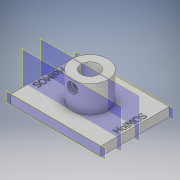
# Autodesk Inventor part: 1.3 Laserhalter_unten
Saved by Autodesk Inventor 2018.3 (Build 223284000, 284)
## iProperties
Created: 2018-11-22
Part Number: 1.3 Laserhalter_unten
Material: Generisch
Document SubType Name: Modeling
Designer: pgmadmin
Density: 1 g/cm^3
Appearance: Vorgabe
Author: pgmadmin
Autodesk Inventor part; units mm, degrees
ref_plane "YZ Plane" through (0, 0, 0) normal (1, 0, 0) x (0, 1, 0)
ref_plane "XY Plane" through (0, 0, 0) normal (0, 0, 1) x (1, 0, 0)
sketch "Skizze1" plane through (0, 0, 0) normal (0, 0, 1) x (1, 0, 0)
  line L0 (-25, -19) -> (25, -19)
  line L1 (25, -19) -> (25, 19)
  line L2 (25, 19) -> (-25, 19)
  line L3 (-25, 19) -> (-25, -19)
  line L4 (-25, -19) -> (25, 19) construction
  line L5 (25, -19) -> (-25, 19) construction
  point P0 (0, 0)
  dimension "d0" = 50
  dimension "d1" = 38
  constraints: 12 end point, 2 midpoint, 2 parallel, 1 horizontal, 1 perpendicular
  measures "d0" distance of L1.end L2.end
  measures "d1" distance of L0.end L1.end
extrude "Extrusion1" add sketch "Skizze1" along normal blind 5
sketch "Skizze2" plane through (0, 0, 5) normal (0, 0, 1) x (1, 0, 0)
  point P0 (0, 0)
ref_plane "Arbeitsebene1" through (0, 19, 0) normal (0, 1, 0) x (-1, 0, 0)
ref_plane "Arbeitsebene2" through (0, -19, 0) normal (0, 1, 0) x (-1, 0, 0)
sketch "Skizze4" plane through (0, 0, 5) normal (0, 0, 1) x (1, 0, 0)
  circle A0 centre (0, 0) radius 10
  circle A1 centre (0, 0) radius 5
  dimension "d12" = 20
  dimension "d13" = 10
  constraints: 2 centre point, 2 coincident
  measures "d12" diameter of A0
  measures "d13" diameter of A1
extrude "Extrusion2" add sketch "Skizze4" along normal blind 15
ref_plane "Arbeitsebene3" through (0, -10, 0) normal (0, 1, 0) x (-1, 0, 0)
sketch "Skizze5" plane through (0, -10, 0) normal (0, 1, 0) x (-1, 0, 0)
  line L0 (10, 20) -> (-10, 20) projected
  point P0 (0, 0)
  point P1 (0, 16)
  dimension "d17" = 4
  measures "d17" distance from line of point (0, 16) L0
hole "Bohrung1" at (0, -10, 16) direction (0, 1, 0) diameter 3 depth 8 tip angle 118 counterbore diameter 5.68 counterbore depth 2
sketch "Skizze6" plane through (0, -10, 0) normal (0, 1, 0) x (-1, 0, 0)
  point P0 (0, 0)
sketch "Skizze7" plane through (0, 0, 0) normal (0, 0, -1) x (-1, 0, 0)
  circle A0 centre (0, 0) radius 2.5
  dimension "d25" = 5
  constraints: 2 coincident, 1 centre point
  measures "d25" diameter of A0
hole "Bohrung2" at (0, 0, 0) direction (0, 0, 1) diameter 5 depth 5 tip angle 118
sketch "Skizze8" plane through (0, 0, 5) normal (0, 0, 1) x (1, 0, 0)
  line L0 (25, 19) -> (-25, 19) projected
  line L1 (-25, -19) -> (25, -19) projected
  line L2 (-24, 19) -> (24, 19)
  line L3 (24, 19) -> (24, -19)
  line L4 (24, -19) -> (-24, -19)
  line L5 (-24, -19) -> (-24, 19)
  line L6 (-25, 19) -> (-25, -19) projected
  line L7 (25, -19) -> (25, 19) projected
  line L8 (-24, 5.3865) -> (-24, 5.8517)
  line L9 (-24, 5.8517) -> (-22.2869, 5.8517)
  line L10 (-22.2869, 5.8517) -> (-22.2869, 7.4627)
  line L11 (-22.2869, 7.4627) -> (-24, 7.4627)
  line L12 (-24, 7.4627) -> (-24, 7.9279)
  line L13 (-24, 7.9279) -> (-20.5, 7.9279)
  line L14 (-20.5, 7.9279) -> (-20.5, 7.4627)
  line L15 (-20.5, 7.4627) -> (-21.8728, 7.4627)
  line L16 (-21.8728, 7.4627) -> (-21.8728, 5.8517)
  line L17 (-21.8728, 5.8517) -> (-20.5, 5.8517)
  line L18 (-20.5, 5.8517) -> (-20.5, 5.3865)
  line L19 (-20.5, 5.3865) -> (-24, 5.3865)
  spline S0 degree 2 poles (-22.6868, 2.5531) (-23.3505, 2.5531) (-24.0737, 3.1912) (-24.0737, 3.7245) knots 0 0 0 1 2 2 2
  spline S1 degree 2 poles (-24.0737, 3.7245) (-24.0737, 4.2719) (-23.3278, 4.8987) (-22.6868, 4.8987) knots 0 0 0 1 2 2 2
  spline S2 degree 2 poles (-22.6868, 4.8987) (-22.0288, 4.8987) (-21.2998, 4.252) (-21.2998, 3.7245) knots 0 0 0 1 2 2 2
  spline S3 degree 2 poles (-21.2998, 3.7245) (-21.2998, 3.1912) (-22.0259, 2.5531) (-22.6868, 2.5531) knots 0 0 0 1 2 2 2
  spline S4 degree 2 poles (-22.6868, 3.0097) (-22.1763, 3.0097) (-21.6799, 3.3813) (-21.6799, 3.7245) knots 0 0 0 1 2 2 2
  spline S5 degree 2 poles (-21.6799, 3.7245) (-21.6799, 4.0677) (-22.1763, 4.4421) (-22.6868, 4.4421) knots 0 0 0 1 2 2 2
  spline S6 degree 2 poles (-22.6868, 4.4421) (-23.1831, 4.4421) (-23.6937, 4.0677) (-23.6937, 3.7245) knots 0 0 0 1 2 2 2
  spline S7 degree 2 poles (-23.6937, 3.7245) (-23.6937, 3.3841) (-23.1917, 3.0097) (-22.6868, 3.0097) knots 0 0 0 1 2 2 2
  line L20 (-24, 1.6483) -> (-24, 2.0908)
  line L21 (-24, 2.0908) -> (-20.344, 2.0908)
  line L22 (-20.344, 2.0908) -> (-20.344, 1.6483)
  line L23 (-20.344, 1.6483) -> (-24, 1.6483)
  line L24 (-24, -2.0361) -> (-24, -1.5709)
  line L25 (-24, -1.5709) -> (-20.985, -1.5709)
  line L26 (-20.985, -1.5709) -> (-23.0357, -0.6576)
  line L27 (-23.0357, -0.6576) -> (-23.0357, -0.374)
  line L28 (-23.0357, -0.374) -> (-20.985, 0.5308)
  line L29 (-20.985, 0.5308) -> (-24, 0.5308)
  line L30 (-24, 0.5308) -> (-24, 0.9648)
  line L31 (-24, 0.9648) -> (-20.5, 0.9648)
  line L32 (-20.5, 0.9648) -> (-20.5, 0.3294)
  line L33 (-20.5, 0.3294) -> (-22.4485, -0.5442)
  line L34 (-22.4485, -0.5442) -> (-20.5, -1.3894)
  line L35 (-20.5, -1.3894) -> (-20.5, -2.0361)
  line L36 (-20.5, -2.0361) -> (-24, -2.0361)
  spline S8 degree 2 poles (-20.8999, -5.2212) (-21.1325, -5.4198) (-21.8132, -5.641) (-22.25, -5.641) knots 0 0 0 1 2 2 2
  spline S9 degree 2 poles (-22.25, -5.641) (-22.6754, -5.641) (-23.3647, -5.4254) (-23.5972, -5.2212) knots 0 0 0 1 2 2 2
  spline S10 degree 2 poles (-23.5972, -5.2212) (-23.8412, -5.0057) (-24.0737, -4.4356) (-24.0737, -4.0924) knots 0 0 0 1 2 2 2
  spline S11 degree 2 poles (-24.0737, -4.0924) (-24.0737, -3.7378) (-23.8327, -3.1706) (-23.5972, -2.9635) knots 0 0 0 1 2 2 2
  spline S12 degree 2 poles (-23.5972, -2.9635) (-23.3647, -2.7622) (-22.6811, -2.5466) (-22.25, -2.5466) knots 0 0 0 1 2 2 2
  spline S13 degree 2 poles (-22.25, -2.5466) (-21.8104, -2.5466) (-21.141, -2.765) (-20.8999, -2.9664) knots 0 0 0 1 2 2 2
  spline S14 degree 2 poles (-20.8999, -2.9664) (-20.6673, -3.1706) (-20.4263, -3.7407) (-20.4263, -4.0924) knots 0 0 0 1 2 2 2
  spline S15 degree 2 poles (-20.4263, -4.0924) (-20.4263, -4.4498) (-20.6759, -5.0227) (-20.8999, -5.2212) knots 0 0 0 1 2 2 2
  spline S16 degree 2 poles (-22.25, -5.156) (-21.904, -5.156) (-21.3679, -5.0057) (-21.1921, -4.8695) knots 0 0 0 1 2 2 2
  spline S17 degree 2 poles (-21.1921, -4.8695) (-21.0105, -4.7305) (-20.829, -4.3391) (-20.829, -4.0952) knots 0 0 0 1 2 2 2
  spline S18 degree 2 poles (-20.829, -4.0952) (-20.829, -3.8428) (-21.0049, -3.4627) (-21.1921, -3.3181) knots 0 0 0 1 2 2 2
  spline S19 degree 2 poles (-21.1921, -3.3181) (-21.3707, -3.1791) (-21.9096, -3.0316) (-22.25, -3.0316) knots 0 0 0 1 2 2 2
  spline S20 degree 2 poles (-22.25, -3.0316) (-22.9392, -3.0316) (-23.671, -3.6102) (-23.671, -4.0952) knots 0 0 0 1 2 2 2
  spline S21 degree 2 poles (-23.671, -4.0952) (-23.671, -4.5802) (-22.9392, -5.156) (-22.25, -5.156) knots 0 0 0 1 2 2 2
  spline S22 degree 2 poles (-24.0624, -7.1272) (-24.0624, -6.7472) (-23.9036, -6.2139) (-23.7901, -5.9785) knots 0 0 0 1 2 2 2
  line L37 (-23.7901, -5.9785) -> (-23.2058, -5.9785)
  line L38 (-23.2058, -5.9785) -> (-23.2058, -6.0126)
  spline S23 degree 2 poles (-23.2058, -6.0126) (-23.4214, -6.2423) (-23.6596, -6.8237) (-23.6596, -7.0932) knots 0 0 0 1 2 2 2
  spline S24 degree 2 poles (-23.6596, -7.0932) (-23.6596, -7.4789) (-23.3391, -7.8732) (-23.0754, -7.8732) knots 0 0 0 1 2 2 2
  spline S25 degree 2 poles (-23.0754, -7.8732) (-22.8655, -7.8732) (-22.6045, -7.6661) (-22.5393, -7.4421) knots 0 0 0 1 2 2 2
  spline S26 degree 2 poles (-22.5393, -7.4421) (-22.4939, -7.2804) (-22.4315, -7.0109) (-22.3805, -6.8096) knots 0 0 0 1 2 2 2
  spline S27 degree 2 poles (-22.3805, -6.8096) (-22.3323, -6.628) (-22.1876, -6.3416) (-22.0713, -6.231) knots 0 0 0 1 2 2 2
  spline S28 degree 2 poles (-22.0713, -6.231) (-21.955, -6.1232) (-21.643, -6.0041) (-21.4388, -6.0041) knots 0 0 0 1 2 2 2
  spline S29 degree 2 poles (-21.4388, -6.0041) (-21.0134, -6.0041) (-20.4376, -6.6677) (-20.4376, -7.1811) knots 0 0 0 1 2 2 2
  spline S30 degree 2 poles (-20.4376, -7.1811) (-20.4376, -7.4761) (-20.5539, -7.998) (-20.6645, -8.222) knots 0 0 0 1 2 2 2
  line L39 (-20.6645, -8.222) -> (-21.2204, -8.222)
  line L40 (-21.2204, -8.222) -> (-21.2204, -8.188)
  spline S31 degree 2 poles (-21.2204, -8.188) (-21.0673, -8.0207) (-20.8404, -7.4988) (-20.8404, -7.2123) knots 0 0 0 1 2 2 2
  spline S32 degree 2 poles (-20.8404, -7.2123) (-20.8404, -6.889) (-21.1438, -6.4891) (-21.3906, -6.4891) knots 0 0 0 1 2 2 2
  spline S33 degree 2 poles (-21.3906, -6.4891) (-21.6118, -6.4891) (-21.8756, -6.7245) (-21.9352, -6.9457) knots 0 0 0 1 2 2 2
  spline S34 degree 2 poles (-21.9352, -6.9457) (-21.9749, -7.0932) (-22.077, -7.5215) (-22.1195, -7.6633) knots 0 0 0 1 2 2 2
  spline S35 degree 2 poles (-22.1195, -7.6633) (-22.2301, -8.0235) (-22.6754, -8.3582) (-23.0016, -8.3582) knots 0 0 0 1 2 2 2
  spline S36 degree 2 poles (-23.0016, -8.3582) (-23.2087, -8.3582) (-23.6058, -8.1908) (-23.7447, -8.0405) knots 0 0 0 1 2 2 2
  spline S37 degree 2 poles (-23.7447, -8.0405) (-23.8979, -7.8732) (-24.0624, -7.4477) (-24.0624, -7.1272) knots 0 0 0 1 2 2 2
  line L41 (24, -5.5814) -> (24, -6.0466)
  line L42 (24, -6.0466) -> (22.2869, -6.0466)
  line L43 (22.2869, -6.0466) -> (22.2869, -7.6576)
  line L44 (22.2869, -7.6576) -> (24, -7.6576)
  line L45 (24, -7.6576) -> (24, -8.1228)
  line L46 (24, -8.1228) -> (20.5, -8.1228)
  line L47 (20.5, -8.1228) -> (20.5, -7.6576)
  line L48 (20.5, -7.6576) -> (21.8728, -7.6576)
  line L49 (21.8728, -7.6576) -> (21.8728, -6.0466)
  line L50 (21.8728, -6.0466) -> (20.5, -6.0466)
  line L51 (20.5, -6.0466) -> (20.5, -5.5814)
  line L52 (20.5, -5.5814) -> (24, -5.5814)
  spline S38 degree 2 poles (22.6868, -2.748) (23.3505, -2.748) (24.0737, -3.3861) (24.0737, -3.9194) knots 0 0 0 1 2 2 2
  spline S39 degree 2 poles (24.0737, -3.9194) (24.0737, -4.4668) (23.3278, -5.0936) (22.6868, -5.0936) knots 0 0 0 1 2 2 2
  spline S40 degree 2 poles (22.6868, -5.0936) (22.0288, -5.0936) (21.2998, -4.4469) (21.2998, -3.9194) knots 0 0 0 1 2 2 2
  spline S41 degree 2 poles (21.2998, -3.9194) (21.2998, -3.3861) (22.0259, -2.748) (22.6868, -2.748) knots 0 0 0 1 2 2 2
  spline S42 degree 2 poles (22.6868, -3.2046) (22.1763, -3.2046) (21.6799, -3.5762) (21.6799, -3.9194) knots 0 0 0 1 2 2 2
  spline S43 degree 2 poles (21.6799, -3.9194) (21.6799, -4.2626) (22.1763, -4.637) (22.6868, -4.637) knots 0 0 0 1 2 2 2
  spline S44 degree 2 poles (22.6868, -4.637) (23.1831, -4.637) (23.6937, -4.2626) (23.6937, -3.9194) knots 0 0 0 1 2 2 2
  spline S45 degree 2 poles (23.6937, -3.9194) (23.6937, -3.579) (23.1917, -3.2046) (22.6868, -3.2046) knots 0 0 0 1 2 2 2
  line L53 (24, -1.8432) -> (24, -2.2857)
  line L54 (24, -2.2857) -> (20.344, -2.2857)
  line L55 (20.344, -2.2857) -> (20.344, -1.8432)
  line L56 (20.344, -1.8432) -> (24, -1.8432)
  line L57 (24, 1.8412) -> (24, 1.376)
  line L58 (24, 1.376) -> (20.985, 1.376)
  line L59 (20.985, 1.376) -> (23.0357, 0.4627)
  line L60 (23.0357, 0.4627) -> (23.0357, 0.1791)
  line L61 (23.0357, 0.1791) -> (20.985, -0.7257)
  line L62 (20.985, -0.7257) -> (24, -0.7257)
  line L63 (24, -0.7257) -> (24, -1.1596)
  line L64 (24, -1.1596) -> (20.5, -1.1596)
  line L65 (20.5, -1.1596) -> (20.5, -0.5243)
  line L66 (20.5, -0.5243) -> (22.4485, 0.3493)
  line L67 (22.4485, 0.3493) -> (20.5, 1.1945)
  line L68 (20.5, 1.1945) -> (20.5, 1.8412)
  line L69 (20.5, 1.8412) -> (24, 1.8412)
  spline S46 degree 2 poles (20.8999, 5.0263) (21.1325, 5.2249) (21.8132, 5.4461) (22.25, 5.4461) knots 0 0 0 1 2 2 2
  spline S47 degree 2 poles (22.25, 5.4461) (22.6754, 5.4461) (23.3647, 5.2306) (23.5972, 5.0263) knots 0 0 0 1 2 2 2
  spline S48 degree 2 poles (23.5972, 5.0263) (23.8412, 4.8108) (24.0737, 4.2407) (24.0737, 3.8975) knots 0 0 0 1 2 2 2
  spline S49 degree 2 poles (24.0737, 3.8975) (24.0737, 3.543) (23.8327, 2.9757) (23.5972, 2.7686) knots 0 0 0 1 2 2 2
  spline S50 degree 2 poles (23.5972, 2.7686) (23.3647, 2.5673) (22.6811, 2.3517) (22.25, 2.3517) knots 0 0 0 1 2 2 2
  spline S51 degree 2 poles (22.25, 2.3517) (21.8104, 2.3517) (21.141, 2.5701) (20.8999, 2.7715) knots 0 0 0 1 2 2 2
  spline S52 degree 2 poles (20.8999, 2.7715) (20.6673, 2.9757) (20.4263, 3.5458) (20.4263, 3.8975) knots 0 0 0 1 2 2 2
  spline S53 degree 2 poles (20.4263, 3.8975) (20.4263, 4.2549) (20.6759, 4.8278) (20.8999, 5.0263) knots 0 0 0 1 2 2 2
  spline S54 degree 2 poles (22.25, 4.9611) (21.904, 4.9611) (21.3679, 4.8108) (21.1921, 4.6746) knots 0 0 0 1 2 2 2
  spline S55 degree 2 poles (21.1921, 4.6746) (21.0105, 4.5357) (20.829, 4.1442) (20.829, 3.9003) knots 0 0 0 1 2 2 2
  spline S56 degree 2 poles (20.829, 3.9003) (20.829, 3.6479) (21.0049, 3.2678) (21.1921, 3.1232) knots 0 0 0 1 2 2 2
  spline S57 degree 2 poles (21.1921, 3.1232) (21.3707, 2.9842) (21.9096, 2.8367) (22.25, 2.8367) knots 0 0 0 1 2 2 2
  spline S58 degree 2 poles (22.25, 2.8367) (22.9392, 2.8367) (23.671, 3.4153) (23.671, 3.9003) knots 0 0 0 1 2 2 2
  spline S59 degree 2 poles (23.671, 3.9003) (23.671, 4.3853) (22.9392, 4.9611) (22.25, 4.9611) knots 0 0 0 1 2 2 2
  spline S60 degree 2 poles (24.0624, 6.9323) (24.0624, 6.5523) (23.9036, 6.019) (23.7901, 5.7836) knots 0 0 0 1 2 2 2
  line L70 (23.7901, 5.7836) -> (23.2058, 5.7836)
  line L71 (23.2058, 5.7836) -> (23.2058, 5.8177)
  spline S61 degree 2 poles (23.2058, 5.8177) (23.4214, 6.0474) (23.6596, 6.6288) (23.6596, 6.8983) knots 0 0 0 1 2 2 2
  spline S62 degree 2 poles (23.6596, 6.8983) (23.6596, 7.284) (23.3391, 7.6783) (23.0754, 7.6783) knots 0 0 0 1 2 2 2
  spline S63 degree 2 poles (23.0754, 7.6783) (22.8655, 7.6783) (22.6045, 7.4712) (22.5393, 7.2472) knots 0 0 0 1 2 2 2
  spline S64 degree 2 poles (22.5393, 7.2472) (22.4939, 7.0855) (22.4315, 6.816) (22.3805, 6.6147) knots 0 0 0 1 2 2 2
  spline S65 degree 2 poles (22.3805, 6.6147) (22.3323, 6.4331) (22.1876, 6.1467) (22.0713, 6.0361) knots 0 0 0 1 2 2 2
  spline S66 degree 2 poles (22.0713, 6.0361) (21.955, 5.9283) (21.643, 5.8092) (21.4388, 5.8092) knots 0 0 0 1 2 2 2
  spline S67 degree 2 poles (21.4388, 5.8092) (21.0134, 5.8092) (20.4376, 6.4729) (20.4376, 6.9862) knots 0 0 0 1 2 2 2
  spline S68 degree 2 poles (20.4376, 6.9862) (20.4376, 7.2812) (20.5539, 7.8031) (20.6645, 8.0271) knots 0 0 0 1 2 2 2
  line L72 (20.6645, 8.0271) -> (21.2204, 8.0271)
  line L73 (21.2204, 8.0271) -> (21.2204, 7.9931)
  spline S69 degree 2 poles (21.2204, 7.9931) (21.0673, 7.8258) (20.8404, 7.3039) (20.8404, 7.0174) knots 0 0 0 1 2 2 2
  spline S70 degree 2 poles (20.8404, 7.0174) (20.8404, 6.6941) (21.1438, 6.2942) (21.3906, 6.2942) knots 0 0 0 1 2 2 2
  spline S71 degree 2 poles (21.3906, 6.2942) (21.6118, 6.2942) (21.8756, 6.5296) (21.9352, 6.7508) knots 0 0 0 1 2 2 2
  spline S72 degree 2 poles (21.9352, 6.7508) (21.9749, 6.8983) (22.077, 7.3266) (22.1195, 7.4684) knots 0 0 0 1 2 2 2
  spline S73 degree 2 poles (22.1195, 7.4684) (22.2301, 7.8286) (22.6754, 8.1633) (23.0016, 8.1633) knots 0 0 0 1 2 2 2
  spline S74 degree 2 poles (23.0016, 8.1633) (23.2087, 8.1633) (23.6058, 7.9959) (23.7447, 7.8456) knots 0 0 0 1 2 2 2
  spline S75 degree 2 poles (23.7447, 7.8456) (23.8979, 7.6783) (24.0624, 7.2528) (24.0624, 6.9323) knots 0 0 0 1 2 2 2
  point P0 (0, 0)
  dimension "d33" = 1
  dimension "d34" = 1
  constraints: 8 end point, 2 parallel, 2 point on line, 2 vertical, 1 horizontal, 1 perpendicular
  measures "d33" distance between parallel lines of L6 L5
  measures "d34" distance between parallel lines of L7 L3
extrude "Extrusion3" cut sketch "Skizze8" against normal blind 2 contours S75 S60 L3 | L3 S60 L70 L71 S61 S62 S63 S64 S65 S66 S67 S68 L72 L73 S69 S70 S71 S72 S73 S74 S75 | L13 L14 L15 L16 L17 L18 L19 L5 L9 L10 L11 | L46 L47 L48 L49 L50 L51 L52 L3 L42 L43 L44 | S48 S49 L3 | L3 S49 S50 S51 S52 S53 S46 S47 S48 | S37 S22 L5 | L5 S22 L37 L38 S23 S24 S25 S26 S27 S28 S29 S30 L39 L40 S31 S32 S33 S34 S35 S36 S37 | L3 L58 L59 L60 L61 L62 L64 L65 L66 L67 L68 L69 | S10 S11 L5 | L5 S11 S12 S13 S14 S15 S8 S9 S10 | S1 S2 S3 S0 L5 | L5 S0 S1 | S39 S40 S41 S38 L3 | L3 S38 S39 | L5 L25 L26 L27 L28 L29 L31 L32 L33 L34 L35 L36 | L21 L22 L23 L5 | L54 L55 L56 L3
